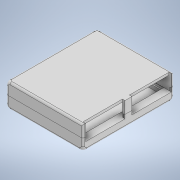
# Autodesk Inventor part: Корпус Unij-A500
Saved by Autodesk Inventor 2022.2 (Build 262287010, 287A)
## iProperties
Created: 2022-09-18
Part Number: Корпус Unij-A500
Material: Типовые
Document SubType Name: Modeling
Designer: Goblin Hero
Density: 1 g/cm^3
Appearance: По умолчанию
Author: Goblin Hero
Autodesk Inventor part; units mm, degrees
ref_plane "YZ Plane" through (0, 0, 0) normal (1, 0, 0) x (0, 1, 0)
ref_plane "XZ Plane" through (0, 0, 0) normal (0, 1, 0) x (-1, 0, 0)
ref_plane "XY Plane" through (0, 0, 0) normal (0, 0, 1) x (1, 0, 0)
sketch "Контур платы" plane through (0, 0, 0) normal (0, 1, 0) x (-1, 0, 0)
  line L0 (-26.25, 33.75) -> (26.25, 33.75)
  line L1 (26.25, 33.75) -> (26.25, -33.75)
  line L2 (26.25, -33.75) -> (-26.25, -33.75)
  line L3 (-26.25, -33.75) -> (-26.25, 33.75)
  line L4 (-26.25, 33.75) -> (26.25, -33.75) construction
  line L5 (26.25, 33.75) -> (-26.25, -33.75) construction
  line L6 (28.25, 35.75) -> (-32.25, 35.75)
  line L7 (-32.25, 35.75) -> (-32.25, -35.75)
  line L8 (-32.25, -35.75) -> (28.25, -35.75)
  line L9 (28.25, -35.75) -> (28.25, 35.75)
  line L10 (26.25, 33.75) -> (28.25, 33.75)
  line L11 (26.25, -33.75) -> (28.25, -33.75)
  circle A0 centre (22.55, 30.05) radius 1.6
  circle A1 centre (22.55, -30.05) radius 1.6
  line L12 (26.25, 32.75) -> (-26.25, 32.75)
  line L13 (26.25, -32.75) -> (-26.25, -32.75)
  line L14 (18.25, -33.75) -> (18.25, -32.75)
  line L15 (-0.25, -33.75) -> (-0.25, -32.75)
  line L16 (26.25, -32.75) -> (19.25, -32.75)
  line L17 (26.25, -25.75) -> (26.25, -32.75)
  line L18 (26.25, 32.75) -> (19.3842, 32.75)
  line L19 (26.25, 32.75) -> (19.25, 32.75)
  line L20 (26.25, 25.75) -> (26.25, 32.75)
  line L21 (26.25, -33.75) -> (19.25, -33.75)
  line L22 (19.25, -33.75) -> (19.25, -26.75)
  line L23 (19.25, -26.75) -> (26.25, -26.75)
  line L24 (26.25, -26.75) -> (26.25, -33.75)
  line L25 (26.25, 33.75) -> (19.25, 33.75)
  line L26 (19.25, 33.75) -> (19.25, 26.75)
  line L27 (19.25, 26.75) -> (26.25, 26.75)
  line L28 (26.25, 26.75) -> (26.25, 33.75)
  point P0 (0, 0)
  point P1 (-2, -35.75)
  point P2 (18.25, -33.25)
  point P3 (-0.25, -33.25)
  dimension "d0" = 52.5
  dimension "d1" = 67.5
  dimension "d3" = 6
  dimension "d4" = 2
  dimension "d5" = 2
  dimension "d6" = 2
  dimension "d7" = 3.2
  dimension "d8" = 3.2
  dimension "d9" = 3.7
  dimension "d10" = 3.7
  dimension "d11" = 3.7
  dimension "d12" = 3.7
  dimension "d13" = 1
  dimension "d14" = 1
  dimension "d15" = 8
  dimension "d19" = 26
  dimension "d30" = 7
  dimension "d31" = 7
  dimension "d32" = 7
  dimension "d33" = 7
  constraints: 58 end point, 10 perpendicular, 10 point on line, 8 parallel, 7 horizontal, 5 midpoint, 2 centre point
  measures "d0" distance of L1.end L2.end
  measures "d1" distance of L0.end L1.end
  measures "d3" distance between parallel lines of L7 L3
  measures "d4" distance between parallel lines of L6 L0
  measures "d5" distance from line of L2 point (-2, -35.75)
  measures "d6" distance between parallel lines of L9 L1
  measures "d7" diameter of A0
  measures "d8" diameter of A1
  measures "d9" distance from line of L0 A0.centre
  measures "d10" distance from line of L1 A0.centre
  measures "d11" distance from line of L2 A1.centre
  measures "d12" distance from line of L1 A1.centre
  measures "d13" distance between parallel lines of L12 L0
  measures "d14" distance between parallel lines of L2 L13
  measures "d15" distance from line of point (18.25, -33.25) L1
  measures "d19" distance from line of L3 point (-0.25, -33.25)
  measures "d30" distance of L22.end L23.end
  measures "d31" distance of L21.end L22.end
  measures "d32" distance of L27.end L26.end
  measures "d33" distance of L26.end L25.end
extrude "Контур по толщине платы" add sketch "Контур платы" along normal blind 1.6 contours L3 L2 L11 L9 L8 L7 L6 L10 L0 | L10 L9 L11 L1
extrude "Пространство под платой" add sketch "Контур платы" against normal blind 3 contours L3 L2 L11 L9 L8 L7 L6 L10 L0 | L0 L26 L12 L3 | L0 L1 L12 L26 | L10 L9 L11 L1 | L12 L1 L27 L26 | L13 L15 L2 L3 | L13 L22 L2 L14 | L2 L22 L13 L1 | L22 L23 L1 L13
sketch "Дно" plane through (0, -3, 0) normal (0, -1, 0) x (1, 0, 0)
  line L0 (-28.25, -35.75) -> (32.25, -35.75) projected
  line L1 (32.25, -35.75) -> (32.25, 35.75) projected
  line L2 (-28.25, -35.75) -> (32.25, -35.75)
  line L3 (32.25, -35.75) -> (32.25, 35.75)
  line L4 (32.25, 35.75) -> (-28.25, 35.75)
  line L5 (-28.25, 35.75) -> (-28.25, -35.75)
  circle A0 centre (-22.55, -30.05) radius 1.6 projected
  circle A1 centre (-22.55, -30.05) radius 2.75
  circle A2 centre (-22.55, 30.05) radius 1.6 projected
  circle A3 centre (-22.55, 30.05) radius 2.75
  point P0 (0, 0)
  dimension "d34" = 5.5
  dimension "d35" = 5.5
  constraints: 8 end point, 2 centre point, 2 coincident, 2 parallel, 1 horizontal, 1 perpendicular
  measures "d34" diameter of A1
  measures "d35" diameter of A3
extrude "Дно корпуса" add sketch "Дно" along normal blind 1.5 contours L5 L4 L1 L0
sketch "Эскиз3" plane through (0, 1.6, 0) normal (0, 1, 0) x (1, 0, 0)
  line L0 (32.25, -35.75) -> (32.25, 35.75) projected
  line L1 (-28.25, -35.75) -> (32.25, -35.75) projected
  line L2 (32.25, 35.75) -> (-28.25, 35.75)
  line L3 (-28.25, 35.75) -> (-28.25, -35.75)
  line L4 (-28.25, -35.75) -> (32.25, -35.75)
  line L5 (32.25, -35.75) -> (32.25, 35.75)
  line L6 (32.25, 34.85) -> (-27.35, 34.85)
  line L7 (-27.35, 34.85) -> (-27.35, -34.85)
  line L8 (-27.35, -34.85) -> (32.25, -34.85)
  line L9 (32.25, 35.75) -> (-28.25, 35.75) projected
  line L10 (15.25, 35.75) -> (15.25, 34.85)
  line L11 (-18.25, 35.75) -> (-18.25, 34.85)
  line L12 (-27.35, 25.75) -> (-28.25, 25.75)
  line L13 (-28.25, -35.75) -> (-28.25, 35.75) projected
  line L14 (-27.35, 13.75) -> (-28.25, 13.75)
  line L15 (-28.25, 35.75) -> (-28.25, -35.75) projected
  line L16 (-27.35, -23.25) -> (-28.25, -23.25)
  line L17 (-27.35, -14.25) -> (-28.25, -14.25)
  line L18 (32.25, 2.75) -> (31.35, 2.75)
  line L19 (31.35, 2.75) -> (31.35, -2.75)
  line L20 (31.35, -2.75) -> (32.25, -2.75)
  line L21 (32.25, -2.75) -> (32.25, 2.75)
  line L22 (32.25, 35.75) -> (31.35, 35.75)
  line L23 (31.35, 35.75) -> (31.35, 33.75)
  line L24 (31.35, 33.75) -> (32.25, 33.75)
  line L25 (32.25, 33.75) -> (32.25, 35.75)
  line L26 (32.25, -35.75) -> (31.35, -35.75)
  line L27 (31.35, -35.75) -> (31.35, -33.75)
  line L28 (31.35, -33.75) -> (32.25, -33.75)
  line L29 (32.25, -33.75) -> (32.25, -35.75)
  point P0 (0, 0)
  point P1 (15.25, 35.3)
  point P2 (-18.25, 35.3)
  point P3 (-27.8, 25.75)
  point P4 (-27.8, 13.75)
  point P5 (-27.8, -23.25)
  point P6 (-27.8, -14.25)
  point P7 (-28.25, 25.75)
  point P8 (-18.25, 35.75)
  point P9 (31.8, 2.75)
  point P10 (31.8, -2.75)
  point P11 (31.35, -34.85)
  point P12 (31.35, 34.85)
  dimension "d36" = 0.9
  dimension "d37" = 0.9
  dimension "d38" = 0.9
  dimension "d39" = 17
  dimension "d40" = 10
  dimension "d41" = 10
  dimension "d42" = 12
  dimension "d43" = 12.5
  dimension "d44" = 9
  dimension "d47" = 33
  dimension "d48" = 33
  dimension "d49" = 0.9
  dimension "d52" = 0.9
  dimension "d53" = 2
  dimension "d54" = 0.9
  dimension "d55" = 2
  constraints: 50 end point, 15 point on line, 11 perpendicular, 8 midpoint, 8 parallel, 5 horizontal, 1 vertical
  measures "d36" distance between parallel lines of L1 L8
  measures "d37" distance between parallel lines of L2 L6
  measures "d38" distance between parallel lines of L3 L7
  measures "d39" distance from line of L5 point (15.25, 35.3)
  measures "d40" distance from line of L3 point (-18.25, 35.3)
  measures "d41" distance from line of L2 point (-27.8, 25.75)
  measures "d42" distance of point (-27.8, 13.75) point (-27.8, 25.75)
  measures "d43" distance from line of L4 point (-27.8, -23.25)
  measures "d44" distance of point (-27.8, -14.25) point (-27.8, -23.25)
  measures "d47" distance from line of L2 point (31.8, 2.75)
  measures "d48" distance from line of L1 point (31.8, -2.75)
  measures "d49" distance between parallel lines of L21 L19
  measures "d52" distance of L24.end L23.end
  measures "d53" distance of L23.end L22.end
  measures "d54" distance of L27.end L28.end
  measures "d55" distance of L26.end L27.end
extrude "Упоры - низ" add sketch "Эскиз3" along normal blind 3 contours L1 L27 L8 L0 | L8 L27 L28 L0 | L1 L3 L16 L7 L8 L27 | L20 L19 L18 L0 | L3 L14 L7 L17 | L24 L23 L6 L0 | L6 L23 L2 L0 | L3 L2 L11 L6 L7 L12 | L6 L10 L2 L23
sketch "Контур крышки" plane through (0, 4.6, 0) normal (0, 1, 0) x (1, 0, 0)
  line L0 (-28.25, -23.25) -> (-28.25, -35.75) projected
  line L1 (-28.25, -35.75) -> (32.25, -35.75)
  line L2 (32.25, -35.75) -> (32.25, 35.75)
  line L3 (32.25, 35.75) -> (-28.25, 35.75)
  line L4 (-28.25, 35.75) -> (-28.25, -35.75)
  line L5 (31.25, 34.75) -> (31.25, -34.75)
  line L6 (31.25, -34.75) -> (-27.25, -34.75)
  line L7 (-27.25, -34.75) -> (-27.25, 34.75)
  line L8 (-27.25, 34.75) -> (31.25, 34.75)
  line L9 (30.25, -33.75) -> (30.25, 33.75)
  line L10 (30.25, 33.75) -> (-26.25, 33.75)
  line L11 (-26.25, 33.75) -> (-26.25, -33.75)
  line L12 (-26.25, -33.75) -> (30.25, -33.75)
  line L13 (15.25, 35.75) -> (15.25, 33.75)
  line L14 (-18.25, 34.85) -> (-18.25, 35.75) projected
  line L15 (-18.25, 35.75) -> (-18.25, 33.75)
  line L16 (-28.25, 35.75) -> (-28.25, 25.75) projected
  line L17 (-28.25, 25.75) -> (-26.25, 25.75)
  line L18 (-28.25, 25.75) -> (-28.25, 13.75) projected
  line L19 (-28.25, 13.75) -> (-26.25, 13.75)
  line L20 (-28.25, 13.75) -> (-28.25, -14.25) projected
  line L21 (-28.25, -14.25) -> (-26.25, -14.25)
  line L22 (-28.25, -23.25) -> (-26.25, -23.25)
  line L23 (31.35, 33.75) -> (32.25, 33.75) projected
  line L24 (30.25, 33.75) -> (32.25, 33.75)
  line L25 (32.25, -33.75) -> (31.35, -33.75) projected
  line L26 (30.25, -33.75) -> (32.25, -33.75)
  line L27 (32.25, -2.75) -> (32.25, 2.75) projected
  line L28 (32.25, 2.75) -> (30.25, 2.75)
  line L29 (32.25, -2.75) -> (30.25, -2.75)
  point P0 (0, 0)
  point P1 (31.25, -2.75)
  point P2 (31.25, 2.75)
  point P3 (31.25, -33.75)
  point P4 (-27.25, -23.25)
  point P5 (-27.25, -14.25)
  point P6 (-27.25, 13.75)
  point P7 (-27.25, 25.75)
  point P8 (-18.25, 34.75)
  point P9 (31.25, 33.75)
  point P10 (15.25, 34.75)
  dimension "d50" = 1
  dimension "d51" = 1
  constraints: 44 end point, 11 perpendicular, 8 point on line, 6 parallel, 1 horizontal, 6 other
  measures "d50" distance between parallel lines of L5 L2
  measures "d51" distance between parallel lines of L5 L9
extrude "Упоры - крышка" add sketch "Контур крышки" against normal blind 2.8 separate body contours L22 L11 L12 L26 L5 L6 L7 | L7 L19 L11 L21 | L7 L8 L15 L10 L11 L17 | L29 L9 L28 L5 | L24 L10 L13 L8 L5
extrude "Боковины крышки" add sketch "Контур крышки" along normal blind 7.5 contours L22 L7 L6 L5 L26 L25 L2 L1 L0 | L4 L19 L7 L21 | L22 L11 L12 L26 L5 L6 L7 | L7 L19 L11 L21 | L4 L3 L14 L15 L8 L7 L17 | L29 L5 L28 L2 | L7 L8 L15 L10 L11 L17 | L29 L9 L28 L5 | L23 L24 L5 L8 L13 L3 L2 | L24 L10 L13 L8 L5 bodies 2
sketch "Крышка" plane through (0, 12.1, 0) normal (0, 1, 0) x (1, 0, 0)
  line L0 (-28.25, -35.75) -> (32.25, -35.75) projected
  line L1 (32.25, 35.75) -> (-28.25, 35.75)
  line L2 (-28.25, 35.75) -> (-28.25, -35.75)
  line L3 (-28.25, -35.75) -> (32.25, -35.75)
  line L4 (32.25, -35.75) -> (32.25, 35.75)
  line L5 (32.25, 35.75) -> (15.25, 35.75) projected
  line L6 (30.25, 35.75) -> (30.25, -35.75)
  line L7 (32.25, 2.75) -> (30.25, 2.75) projected
  line L8 (32.25, 2.75) -> (30.25, 2.75)
  line L9 (32.25, -2.75) -> (32.25, 2.75) projected
  line L10 (30.25, 2.75) -> (30.25, -2.75) projected
  line L11 (32.25, -2.75) -> (30.25, -2.75)
  line L12 (15.25, 33.75) -> (32.25, 33.75) projected
  line L13 (32.25, 33.75) -> (30.25, 33.75)
  line L14 (32.25, -33.75) -> (-26.25, -33.75) projected
  line L15 (30.25, -33.75) -> (32.25, -33.75)
  line L16 (30.25, 33.75) -> (-26.25, 33.75)
  line L17 (-26.25, -33.75) -> (-26.25, -23.25) projected
  line L18 (-26.25, 33.75) -> (-26.25, -33.75)
  line L19 (-26.25, -33.75) -> (30.25, -33.75)
  line L20 (15.25, 35.75) -> (15.25, 33.75) projected
  line L21 (15.25, 35.75) -> (15.25, 33.75)
  line L22 (-18.25, 35.75) -> (-28.25, 35.75) projected
  line L23 (-18.25, 35.75) -> (-18.25, 33.75)
  line L24 (-28.25, 35.75) -> (-28.25, 25.75) projected
  line L25 (-28.25, 25.75) -> (-26.25, 25.75) projected
  line L26 (-28.25, 25.75) -> (-26.25, 25.75)
  line L27 (-27.25, 13.75) -> (-28.25, 13.75) projected
  line L28 (-26.25, 13.75) -> (-28.25, 13.75) projected
  line L29 (-28.25, 13.75) -> (-26.25, 13.75)
  line L30 (0.25, 35.75) -> (0.25, 33.75)
  line L31 (-28.25, 17.25) -> (-26.25, 17.25)
  line L32 (-26.25, -23.25) -> (-28.25, -23.25) projected
  line L33 (-26.25, -23.25) -> (-28.25, -23.25)
  line L34 (-28.25, -14.25) -> (-27.25, -14.25) projected
  line L35 (-26.25, -14.25) -> (-28.25, -14.25)
  line L36 (-26.25, -33.75) -> (-19.25, -33.75)
  line L37 (-19.25, -33.75) -> (-19.25, -26.75)
  line L38 (-19.25, -26.75) -> (-26.25, -26.75)
  line L39 (-26.25, -26.75) -> (-26.25, -33.75)
  line L40 (-26.25, 33.75) -> (-26.25, 25.75) projected
  line L41 (-19.25, 26.75) -> (-26.25, 26.75) projected
  line L42 (-26.25, 33.75) -> (-19.25, 33.75)
  line L43 (-19.25, 33.75) -> (-19.25, 26.75)
  line L44 (-19.25, 26.75) -> (-26.25, 26.75)
  line L45 (-26.25, 26.75) -> (-26.25, 33.75)
  circle A0 centre (-22.55, 30.05) radius 1.6 projected
  circle A1 centre (-22.55, 30.05) radius 0.75
  circle A2 centre (-22.55, -30.05) radius 1.6 projected
  circle A3 centre (-22.55, -30.05) radius 0.75
  point P0 (0, 0)
  point P1 (32.25, -35.75)
  point P2 (0.25, 34.75)
  point P3 (-27.25, 17.25)
  dimension "d60" = 2
  dimension "d63" = 18.5
  dimension "d64" = 8.5
  dimension "d71" = 1.5
  dimension "d72" = 1.5
  constraints: 56 end point, 10 point on line, 8 collinear, 8 perpendicular, 6 parallel, 4 horizontal, 2 centre point, 2 coincident, 2 midpoint
  measures "d60" distance between parallel lines of L4 L6
  measures "d63" distance from line of point (0.25, 34.75) L23
  measures "d64" distance from line of point (-27.25, 17.25) L25
  measures "d71" diameter of A1
  measures "d72" diameter of A3
extrude "Верхняя крышка" add sketch "Крышка" along normal blind 2 contours L2 L32 L17 L14 L6 L0 | L6 L14 L4 L0 | L2 L34 L35 L18 L32 | L14 L37 L38 L17 L18 L41 L43 L16 L12 L6 | L2 L27 L28 L18 L35 L34 | L6 L7 L4 L11 | L14 L17 L38 L37 | L2 L31 L18 L28 L27 | L2 L25 L18 L31 | L12 L20 L1 L6 | L6 L1 L4 L12 | L2 L1 L23 L16 L18 L25 | L16 L30 L1 L20 | L16 L23 L1 L30 | L18 L16 L43 L41 | A0 | A1 | A2 | A3 bodies 2
extrude "Над кнопками" add sketch "Крышка" against normal blind 3 contours L2 L25 L18 L31 | L16 L23 L1 L30 bodies 2
extrude "Над диодами" add sketch "Крышка" against normal blind 7.5 contours L2 L31 L18 L28 L27 | L16 L30 L1 L20 bodies 2
extrude "Над USB" add sketch "Крышка" against normal blind 6.5 contours L2 L34 L35 L18 L32 bodies 2
extrude "Бочонки под саморезы" add sketch "Крышка" against normal blind 10.3 contours L14 L17 L38 L37 | L18 L16 L43 L41 | A0 | A2 bodies 2
fillet "Сопряжение1" radius 1.5 15 edges at (2, -4.5, 35.75) (32.25, -4.5, 0) (32.25, 0.05, 35.75) (-28.25, 0.05, 35.75) (32.25, 0.05, -35.75) (2, -4.5, -35.75) (-28.25, 0.05, -35.75) (-28.25, -4.5, 0) (32.25, 9.35, 35.75) (2, 14.1, 35.75) (-28.25, 9.35, 35.75) (32.25, 9.35, -35.75) (2, 14.1, -35.75) (-28.25, 9.35, -35.75) (-28.25, 14.1, 0)
